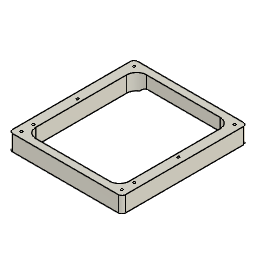
Base Stand - Compact (Autodesk Fusion 360 design; units mm, degrees)
Autodesk Fusion 360 part; units mm, degrees
sketch "Sketch1" plane through (0, 0, 0) normal (0, 0, 1) x (1, 0, 0)
  line L0 (-92.5, 102.5) -> (92.5, 102.5)
  line L1 (92.5, 102.5) -> (92.5, -102.5)
  line L2 (92.5, -102.5) -> (-92.5, -102.5)
  line L3 (-92.5, -102.5) -> (-92.5, 102.5)
  line L4 (-76.5, 90.5) -> (76.5, 90.5)
  line L5 (76.5, 90.5) -> (76.5, -90.5)
  line L6 (76.5, -90.5) -> (-76.5, -90.5)
  line L7 (-76.5, -90.5) -> (-76.5, 90.5)
  dimension "d5" = 185
  dimension "d6" = 92.5
  dimension "d7" = 205
  dimension "d8" = 102.5
  dimension "d9" = 16
  dimension "d10" = 12
  dimension "d11" = 16
  dimension "d12" = 12
  constraint horizontal L0
  constraint vertical L1
  constraint horizontal L2
  constraint vertical L3
  constraint horizontal L4
  constraint vertical L5
  constraint horizontal L6
  constraint vertical L7
  measures "d5" distance of L1.end L2.end
  measures "d6" distance of origin L3
  measures "d7" distance of L0.start L2.end
  measures "d8" distance of origin L0
  measures "d9" distance of L1 L5
  measures "d10" distance of L2 L6
  measures "d11" distance of L3 L7
  measures "d12" distance of L0 L4
extrude "Extrude1" add sketch "Sketch1" against normal blind 36
sketch "Sketch2" plane through (92.5, 0, 0) normal (1, 0, 0) x (0, 1, 0)
  line L0 (102.5, 0) -> (-102.5, 0)
  line L1 (-102.5, 0) -> (-102.5, -36)
  line L2 (-102.5, -36) -> (102.5, -36)
  line L3 (102.5, -36) -> (102.5, 0)
  line L4 (-82.5, -36) -> (82.5, -36)
  line L5 (82.5, -36) -> (82.5, -26)
  line L6 (82.5, -26) -> (-82.5, -26)
  line L7 (-82.5, -26) -> (-82.5, -36)
  dimension "d15" = 10
  dimension "d16" = 20
  dimension "d17" = 20
  constraint horizontal L4
  constraint vertical L5
  constraint horizontal L6
  constraint vertical L7
  constraint coincident L2 L4.start
  measures "d15" distance of L4 L6
  measures "d16" distance of L3 L5
  measures "d17" distance of L1 L7
extrude "Extrude2" cut sketch "Sketch2" against normal up to surface (185 mm away) contours L2 L4 L5 L6 L7
sketch "Sketch3" plane through (0, -102.5, 0) normal (0, -1, 0) x (1, 0, 0)
  line L0 (92.5, 0) -> (-92.5, 0)
  line L1 (-92.5, 0) -> (-92.5, -36)
  line L2 (-92.5, -36) -> (92.5, -36)
  line L3 (92.5, -36) -> (92.5, 0)
  line L4 (-72.5, -26) -> (72.5, -26)
  line L5 (72.5, -26) -> (72.5, -36)
  line L6 (72.5, -36) -> (-72.5, -36)
  line L7 (-72.5, -36) -> (-72.5, -26)
  dimension "d20" = 10
  dimension "d21" = 20
  dimension "d22" = 20
  constraint horizontal L4
  constraint vertical L5
  constraint horizontal L6
  constraint vertical L7
  constraint coincident L2 L5.end
  measures "d20" distance of L4 L6
  measures "d21" distance of L3 L5
  measures "d22" distance of L1 L7
extrude "Extrude3" cut sketch "Sketch3" against normal blind 12 contours L2 L4 L5 L6 L7
fillet "Fillet1" radius 16 4 edges at (-76.5, 90.5, -18) (76.5, 90.5, -18) (76.5, -90.5, -18) (-76.5, -90.5, -18)
sketch "Sketch4" plane through (0, 0, 0) normal (0, 0, 1) x (-1, 0, 0)
  line L0 (-60.5, 90.5) -> (60.5, 90.5)
  arc A0 (76.5, 74.5) -> (60.5, 90.5) centre (60.5, 74.5) ccw
  line L1 (76.5, 74.5) -> (76.5, -74.5)
  arc A1 (60.5, -90.5) -> (76.5, -74.5) centre (60.5, -74.5) ccw
  line L2 (60.5, -90.5) -> (-60.5, -90.5)
  arc A2 (-76.5, -74.5) -> (-60.5, -90.5) centre (-60.5, -74.5) ccw
  line L3 (-76.5, -74.5) -> (-76.5, 74.5)
  arc A3 (-60.5, 90.5) -> (-76.5, 74.5) centre (-60.5, 74.5) ccw
  line L4 (92.5, 102.5) -> (-92.5, 102.5)
  line L5 (-92.5, 102.5) -> (-92.5, -102.5)
  line L6 (-92.5, -102.5) -> (92.5, -102.5)
  line L7 (92.5, -102.5) -> (92.5, 102.5)
  line L8 (92.5, -92.5) -> (-92.5, -92.5) construction
  line L9 (92.5, 92.5) -> (-92.5, 92.5) construction
  line L10 (82.5, -102.5) -> (82.5, 102.5) construction
  line L11 (-82.5, -102.5) -> (-82.5, 102.5) construction
  circle A4 centre (82.5, -92.5) radius 1.9
  circle A5 centre (-82.5, -92.5) radius 1.9
  circle A6 centre (82.5, 92.5) radius 1.9
  circle A7 centre (-82.5, 92.5) radius 1.9
  line L12 (103.0848, 0) -> (-103.0848, 0) construction
  circle A8 centre (82.5, 0) radius 1.9
  circle A9 centre (-82.5, 0) radius 1.9
  circle A10 centre (82.5, 72.5) radius 1.9
  circle A11 centre (-82.5, 72.5) radius 1.9
  line L13 (113.4031, 72.5) -> (-110.5504, 72.5) construction
  dimension "d26" = 10
  dimension "d27" = 10
  dimension "d28" = 10
  dimension "d29" = 10
  dimension "d31" = 3.8
  dimension "d32" = 3.8
  dimension "d33" = 3.8
  dimension "d34" = 3.8
  dimension "d706" = 3.8
  dimension "d707" = 3.8
  dimension "d910" = 3.8
  dimension "d911" = 3.8
  dimension "d912" = 20
  constraint coincident L7 L8.start
  constraint coincident L5 L8.end
  constraint perpendicular L5 L8
  constraint coincident L7 L9.start
  constraint coincident L5 L9.end
  constraint perpendicular L5 L9
  constraint coincident L6 L10.start
  constraint coincident L4 L10.end
  constraint perpendicular L4 L10
  constraint coincident L6 L11.start
  constraint coincident L4 L11.end
  constraint perpendicular L4 L11
  constraint coincident L10 A4.centre
  constraint coincident L8 A4.centre
  constraint coincident L8 A5.centre
  constraint coincident L11 A5.centre
  constraint coincident L9 A6.centre
  constraint coincident L10 A6.centre
  constraint coincident L9 A7.centre
  constraint coincident L11 A7.centre
  constraint perpendicular L5 L12
  constraint midpoint origin L12
  constraint midpoint L10 A8.centre
  constraint midpoint L11 A9.centre
  constraint coincident L10 A10.centre
  constraint coincident L11 A11.centre
  constraint perpendicular L11 L13
  constraint coincident A10.centre L13
  constraint coincident A11.centre L13
  measures "d26" distance of L7 L10
  measures "d27" distance of L5 L11
  measures "d28" distance of L4 L9
  measures "d29" distance of L6 L8
  measures "d31" diameter of A4
  measures "d32" diameter of A5
  measures "d33" diameter of A6
  measures "d34" diameter of A7
  measures "d706" diameter of A8
  measures "d707" diameter of A9
  measures "d910" diameter of A10
  measures "d911" diameter of A11
  measures "d912" distance of A6.centre L13
extrude "Extrude8" cut sketch "Sketch4" against normal through all contours A10 | A11
extrude "Extrude6" cut sketch "Sketch4" against normal through all contours A8 | A9
extrude "Extrude4" cut sketch "Sketch4" against normal up to surface (36 mm away) contours A4 | A5 | A6 | A7
sketch "Sketch5" plane through (0, 102.5, 0) normal (0, 1, 0) x (-1, 0, 0)
  line L0 (92.5, 0) -> (-92.5, 0)
  line L1 (-92.5, 0) -> (-92.5, -36)
  line L2 (-92.5, -36) -> (92.5, -36)
  line L3 (92.5, -36) -> (92.5, 0)
  line L4 (-72.5, -36) -> (72.5, -36)
  line L5 (72.5, -36) -> (72.5, -20)
  line L6 (72.5, -20) -> (-72.5, -20)
  line L7 (-72.5, -20) -> (-72.5, -36)
  dimension "d39" = 20
  dimension "d40" = 20
  dimension "d41" = 16
  constraint horizontal L4
  constraint vertical L5
  constraint horizontal L6
  constraint vertical L7
  constraint coincident L2 L4.start
  measures "d39" distance of L3 L5
  measures "d40" distance of L1 L7
  measures "d41" distance of L4 L6
extrude "Extrude5" cut sketch "Sketch5" against normal blind 40 contours L2 L4 L5 L6 L7
fillet "Fillet2" radius 10 6 edges at (83.4282, -82.5, -26) (-83.4282, -82.5, -26) (-72.5, -93.7915, -26) (72.5, -93.7915, -26) (83.4282, 82.5, -26) (-83.4282, 82.5, -26)
fillet "Fillet2" radius 16 2 edges at (72.5, 93.7915, -20) (-72.5, 93.7915, -20)
fillet "Fillet3" radius 6 2 edges at (92.5, 102.5, -18) (-92.5, 102.5, -18)
fillet "Fillet3" radius 6 2 edges at (92.5, -102.5, -18) (-92.5, -102.5, -18)
ref_plane "WorkPlane1" through (0, 97, 0) normal (0, 1, 0) x (0, 0, 1)
sketch "Sketch6" plane through (0, 97, 0) normal (0, 1, 0) x (1, 0, 0)
  line L0 (99.0072, 20) -> (-99.0626, 20) construction
  circle A0 centre (42.4387, 20) radius 6
  line L1 (56.5, 20) -> (-56.5, 20)
  dimension "d770" = 12
  constraint horizontal L0
  constraint coincident L0 A0.centre
  constraint collinear L0 L1
  measures "d770" diameter of A0
pipe "Pipe1" cut diameter 6 path "Sketch6" along A0
pattern_linear "R-Pattern1" count 1 spacing 0 along (0, 0, 1) count 5 spacing 20 along (-1, 0, 0) of "Pipe1"
sketch "Sketch10" plane through (92.5, 0, 0) normal (1, 0, 0) x (0, 1, 0)
  line L0 (-96.5, 0) -> (-96.5, -36)
  line L1 (-96.5, -36) -> (-82.5, -36)
  arc A0 (-72.5, -26) -> (-82.5, -36) centre (-72.5, -36) ccw
  line L2 (-72.5, -26) -> (72.5, -26)
  arc A1 (82.5, -36) -> (72.5, -26) centre (72.5, -36) ccw
  line L3 (82.5, -36) -> (96.5, -36)
  line L4 (96.5, -36) -> (96.5, 0)
  line L5 (96.5, 0) -> (-96.5, 0)
  line L6 (-110, -26) -> (110, -26)
  line L7 (110, -26) -> (110, -38)
  line L8 (110, -38) -> (-110, -38)
  line L9 (-110, -38) -> (-110, -26)
  point P0 (0, -38)
  dimension "d1328" = 220
  dimension "d1329" = 12
  constraint horizontal L6
  constraint vertical L7
  constraint horizontal L8
  constraint vertical L9
  constraint collinear L2 L6
  constraint midpoint L8 P0
  constraint vertical origin P0
  measures "d1328" distance of L7 L9
  measures "d1329" distance of L6.start L8.end
extrude "Extrude10" cut sketch "Sketch10" against normal through all contours L0 L1 A0 L6 | L0 L1 A0 L2 A1 L3 L4 L6 L7 L8 L9 | A1 L3 L4 L6
equation "d6 = d5 / 2"
equation "d8 = d7 / 2"
equation "d27 = d26"
equation "d28 = d26"
equation "d29 = d26"
equation "d32 = d31"
equation "d33 = d31"
equation "d34 = d31"
equation "d706 = d31"
equation "d707 = d31"
equation "d910 = d33"
equation "d911 = d34"
